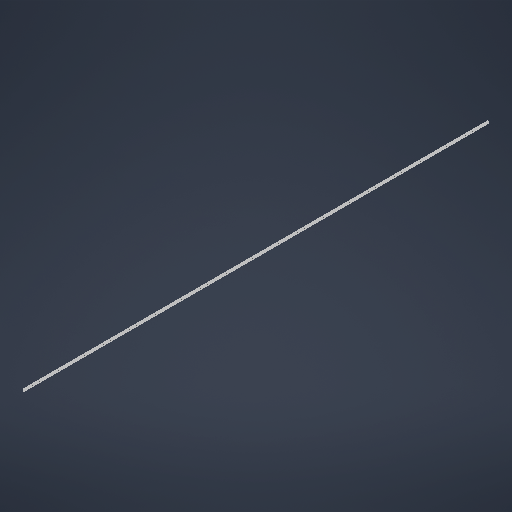
# Autodesk Inventor part: SP40-02 JUNTA
Saved by Autodesk Inventor 2025 (Build 290162000, 162)
## iProperties
Created: 2026-01-18
Part Number: SP40-02 JUNTA
Material: Plástico ABS
Document SubType Name: Modeling
Designer: ROLANDO
Density: 1.06 g/cm^3
Appearance: Gris oscuro
Author: ROLANDO
Autodesk Inventor part; units mm, degrees
ref_plane "YZ Plane" through (0, 0, 0) normal (1, 0, 0) x (0, 1, 0)
ref_plane "XZ Plane" through (0, 0, 0) normal (0, 1, 0) x (-1, 0, 0)
ref_plane "XY Plane" through (0, 0, 0) normal (0, 0, 1) x (1, 0, 0)
sketch "Boceto1" plane through (0, 0, 0) normal (0, 0, 1) x (1, 0, 0)
  line L0 (24.7, 53.7) -> (24.7, 53.26)
  line L1 (28.5, 53.7) -> (28.5, 47.2)
  line L2 (24.7, 47.2) -> (24.7, 47.24)
  line L3 (26.1, 47.2) -> (28.5, 47.2)
  line L4 (26.1, 48.25) -> (25.3942, 48.25)
  line L5 (25.3942, 48.25) -> (24.7, 47.24)
  line L6 (26.1, 52.25) -> (25.3942, 52.25)
  line L7 (26.1, 53.7) -> (28.5, 53.7)
  line L8 (24.7, 53.26) -> (25.3942, 52.25)
  line L9 (26.1, 53.7) -> (26.1, 52.25)
  line L10 (26.1, 47.2) -> (26.1, 48.25)
  line L11 (24.7, 53.26) -> (24.7, 47.2)
  point P0 (28.5, 50.45)
  dimension "d78" = 6.5
  dimension "d84" = 1.4
  dimension "d88" = 2.4
  dimension "d95" = 6.02
  dimension "d99" = 111
  dimension "d100" = 2.4
  dimension "d108" = 4
  dimension "d109" = 0.7058
  dimension "d110" = 0.7058
  constraints: 24 end point, 3 point on line, 2 equal length, 2 horizontal, 2 vertical, 1 midpoint
  measures "d78" distance between parallel lines of L3 L7
  measures "d84" distance between parallel lines of L2 L10
  measures "d88" distance between parallel lines of L1 L9
  measures "d95" distance of L2.end L0.end
  measures "d99" angle of L5 L8
  measures "d100" distance between parallel lines of L1 L10
  measures "d108" distance between parallel lines of L4 L6
  measures "d109" distance of L6.start L6.end
  measures "d110" distance of L4.start L4.end
extrude "Extrusión1" add sketch "Boceto1" against normal blind 2100
